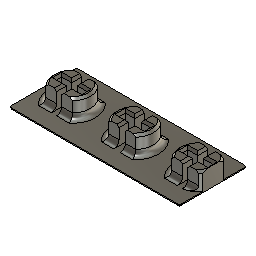
iNTEX_2u_Rotated (Autodesk Fusion 360 design; units mm, degrees)
Autodesk Fusion 360 part; units mm, degrees
sketch "Sketch1" plane through (0, 0, 0) normal (0, 0, 1) x (1, 0, 0)
  line L0 (18.5, 9) -> (-18.5, 9) construction
  line L1 (-18.5, 9) -> (-18.5, -9) construction
  line L2 (-18.5, -9) -> (18.5, -9) construction
  line L3 (18.5, -9) -> (18.5, 9) construction
  line L4 (18.5, 9) -> (-18.5, -9) construction
  line L5 (-18.5, 9) -> (18.5, -9) construction
  line L6 (-17.5, 6.4) -> (14.9, 6.4)
  line L7 (14.9, 6.4) -> (14.9, -6.4)
  line L8 (14.9, -6.4) -> (-17.5, -6.4)
  line L9 (-17.5, -6.4) -> (-17.5, 6.4)
  circle A0 centre (0, 0) radius 3.5
  line L10 (2.4, -0.6) -> (-2.4, -0.6)
  line L11 (-2.4, -0.6) -> (-2.4, 0.6)
  line L12 (-2.4, 0.6) -> (2.4, 0.6)
  line L13 (2.4, 0.6) -> (2.4, -0.6)
  line L14 (2.4, -0.6) -> (-2.4, 0.6) construction
  line L15 (-2.4, -0.6) -> (2.4, 0.6) construction
  line L16 (0.6, -2.4) -> (-0.6, -2.4)
  line L17 (-0.6, -2.4) -> (-0.6, 2.4)
  line L18 (-0.6, 2.4) -> (0.6, 2.4)
  line L19 (0.6, 2.4) -> (0.6, -2.4)
  line L20 (0.6, -2.4) -> (-0.6, 2.4) construction
  line L21 (-0.6, -2.4) -> (0.6, 2.4) construction
  line L22 (-0.6, 2.4) -> (-2.5475, 2.4)
  line L23 (0.6, 2.4) -> (2.5475, 2.4)
  line L24 (-0.6, -2.4) -> (-2.5475, -2.4)
  line L25 (0.6, -2.4) -> (2.5475, -2.4)
  line L26 (0, 0) -> (0, 6.2895) construction
  line L27 (0, 0) -> (12, 0) construction
  circle A1 centre (12, 0) radius 3.5
  line L28 (14.4, -0.5) -> (9.6, -0.5)
  line L29 (9.6, -0.5) -> (9.6, 0.5)
  line L30 (9.6, 0.5) -> (14.4, 0.5)
  line L31 (14.4, 0.5) -> (14.4, -0.5)
  line L32 (14.4, -0.5) -> (9.6, 0.5) construction
  line L33 (9.6, -0.5) -> (14.4, 0.5) construction
  line L34 (12.5, -2.4) -> (11.5, -2.4)
  line L35 (11.5, -2.4) -> (11.5, 2.4)
  line L36 (11.5, 2.4) -> (12.5, 2.4)
  line L37 (12.5, 2.4) -> (12.5, -2.4)
  line L38 (12.5, -2.4) -> (11.5, 2.4) construction
  line L39 (11.5, -2.4) -> (12.5, 2.4) construction
  line L40 (11.5, 2.4) -> (9.4525, 2.4)
  line L41 (12.5, 2.4) -> (14.5475, 2.4)
  line L42 (11.5, -2.4) -> (9.4525, -2.4)
  line L43 (12.5, -2.4) -> (14.5475, -2.4)
  circle A2 centre (-12, 0) radius 3.5
  line L44 (-11.5, 2.4) -> (-9.4525, 2.4)
  line L45 (-11.5, 2.4) -> (-12.5, 2.4)
  line L46 (-12.5, 2.4) -> (-14.5475, 2.4)
  line L47 (-11.5, -2.4) -> (-9.4525, -2.4)
  line L48 (-12.5, -2.4) -> (-11.5, -2.4)
  line L49 (-12.5, -2.4) -> (-14.5475, -2.4)
  line L50 (-11.5, -2.4) -> (-11.5, 2.4)
  line L51 (-12.5, 2.4) -> (-12.5, -2.4)
  line L52 (-14.4, -0.5) -> (-9.6, -0.5)
  line L53 (-9.6, 0.5) -> (-14.4, 0.5)
  line L54 (-14.4, 0.5) -> (-14.4, -0.5)
  line L55 (-9.6, -0.5) -> (-9.6, 0.5)
  point P0 (12, 0)
  point P1 (12, 0)
  dimension "d1" = 37
  dimension "d2" = 18
  dimension "d3" = 2.6
  dimension "d4" = 2.6
  dimension "d5" = 3.6
  dimension "d6" = 1
  dimension "d7" = 7
  dimension "d8" = 4.8
  dimension "d9" = 1.2
  dimension "d10" = 1.2
  dimension "d11" = 4.8
  dimension "d19" = 12
  dimension "d20" = 7
  dimension "d21" = 4.8
  dimension "d22" = 1
  dimension "d23" = 4.8
  dimension "d24" = 1
  constraint perpendicular L0 L1
  constraint parallel L0 L2
  constraint parallel L1 L3
  constraint horizontal L0
  constraint coincident L4 A0.centre
  constraint coincident L5 A0.centre
  constraint coincident A0.centre L26.start
  constraint horizontal L6
  constraint vertical L7
  constraint horizontal L8
  constraint vertical L9
  constraint perpendicular L10 L11
  constraint parallel L10 L12
  constraint parallel L11 L13
  constraint horizontal L10
  constraint coincident L14 A0.centre
  constraint coincident L15 A0.centre
  constraint perpendicular L16 L17
  constraint parallel L16 L18
  constraint parallel L17 L19
  constraint horizontal L16
  constraint coincident L20 A0.centre
  constraint coincident L21 A0.centre
  constraint coincident A0 L22.end
  constraint perpendicular L17 L22
  constraint coincident A0 L23.end
  constraint perpendicular L19 L23
  constraint coincident A0 L24.end
  constraint perpendicular L17 L24
  constraint coincident A0 L25.end
  constraint perpendicular L19 L25
  constraint vertical L26
  constraint perpendicular L19 L27
  constraint coincident P1 P0
  constraint perpendicular L28 L29
  constraint parallel L28 L30
  constraint parallel L29 L31
  constraint horizontal L28
  constraint coincident L32 P1
  constraint coincident L33 P1
  constraint perpendicular L34 L35
  constraint parallel L34 L36
  constraint parallel L35 L37
  constraint horizontal L34
  constraint coincident L38 P1
  constraint coincident L39 P1
  constraint coincident A1 L40.end
  constraint perpendicular L35 L40
  constraint coincident A1 L41.end
  constraint perpendicular L37 L41
  constraint coincident A1 L42.end
  constraint perpendicular L35 L42
  constraint coincident A1 L43.end
  constraint perpendicular L37 L43
  constraint symmetric L26 A1 A2
  constraint symmetric L26 L28.start L52.start
  constraint symmetric L26 L28.end L52.end
  constraint symmetric L26 L29.end L53.start
  constraint symmetric L26 L30.end L53.end
  constraint symmetric L26 L34.start L48.start
  constraint symmetric L26 L34.end L47.start
  constraint symmetric L26 L35.end L44.start
  constraint symmetric L26 L36.end L45.end
  constraint symmetric L26 L40.end L44.end
  constraint symmetric L26 L41.end L46.end
  constraint symmetric L26 L42.end L47.end
  constraint symmetric L26 L43.end L49.end
  measures "d1" distance of L1.end L2.end
  measures "d2" distance of L0.end L1.end
  measures "d3" distance of L2 L8
  measures "d4" distance of L0 L6
  measures "d5" distance of L3 L7
  measures "d6" distance of L1 L9
  measures "d7" diameter of A0
  measures "d8" distance of L11.end L12.end
  measures "d9" distance of L10.end L11.end
  measures "d10" distance of L17.end L18.end
  measures "d11" distance of L16.end L17.end
  measures "d19" distance of A0.centre P1
  measures "d20" diameter of A1
  measures "d21" distance of L29.end L30.end
  measures "d22" distance of L28.end L29.end
  measures "d23" distance of L34.end L35.end
  measures "d24" distance of L35.end L36.end
extrude "Extrude1" add sketch "Sketch1" along normal blind 0.6 contours L6 L7 L8 L9 A1 | L7 A1 L28 L30 L31 L37 L41 L43 | A1 L36 L40 L41 | A1 L34 L42 L43 | A1 L28 L29 L30 L35 L40 L42 | L30 L35 L36 L37 | L28 L34 L35 L37 | L28 L30 L35 L37 | L28 L30 L31 L37 | L28 L29 L30 L35 | A0 L10 L12 L13 L19 L23 L25 | A0 L18 L22 L23 | A0 L16 L24 L25 | A0 L10 L11 L12 L17 L22 L24 | L12 L17 L18 L19 | L10 L16 L17 L19 | L10 L12 L17 L19 | L10 L12 L13 L19 | L10 L11 L12 L17 | A2 L44 L47 L50 L52 L53 L55 | A2 L44 L45 L46 | A2 L47 L48 L49 | A2 L46 L49 L51 L52 L53 L54 | L45 L50 L51 L53 | L48 L50 L51 L52 | L50 L52 L53 L55 | L50 L51 L52 L53 | L51 L52 L53 L54
extrude "Extrude2" add sketch "Sketch1" along normal blind 4 contours L7 A1 L28 L30 L31 L37 L41 L43 | A1 L28 L29 L30 L35 L40 L42 | A0 L10 L12 L13 L19 L23 L25 | A0 L10 L11 L12 L17 L22 L24 | A2 L44 L47 L50 L52 L53 L55 | A2 L46 L49 L51 L52 L53 L54
fillet "Fillet1" radius 1 17 edges at (-1.5738, -2.4, 0.6) (-3.5, 0, 0.6) (1.5738, -2.4, 0.6) (3.5, 0, 0.6) (1.5738, 2.4, 0.6) (-1.5738, 2.4, 0.6) (-10.4762, 2.4, 0.6) (-8.5, 0, 0.6) (-13.5238, 2.4, 0.6) (-15.5, 0, 0.6) (8.5, 0, 0.6) (10.4762, 2.4, 0.6) (13.5238, 2.4, 0.6) (-13.5238, -2.4, 0.6) (-10.4762, -2.4, 0.6) (10.4762, -2.4, 0.6) (13.5238, -2.4, 0.6)
fillet "Fillet1" radius 0.5 4 edges at (14.9, 6.4, 0.3) (-17.5, 6.4, 0.3) (14.9, -6.4, 0.3) (-17.5, -6.4, 0.3)
chamfer "Chamfer1" distance 0.4 angle 45 45 edges at (-1.3, 6.4, 0) (-17.3536, 6.2536, 0) (-17.5, 0, 0) (-17.3536, -6.2536, 0) (-1.3, -6.4, 0) (14.7536, -6.2536, 0) (14.9, 0, 0) (14.7536, 6.2536, 0) (-0.6, 1.5, 4) (-1.5, 0.6, 4) (-2.4, 0, 4) (-1.5, -0.6, 4) (-0.6, -1.5, 4) (0.6, -1.5, 4) (1.5, -0.6, 4) (2.4, 0, 4) (1.5, 0.6, 4) (0.6, 1.5, 4) (3.5, 0, 4) (-3.5, 0, 4) (-12.5, -1.45, 4) (-13.45, -0.5, 4) (-14.4, 0, 4) (-13.45, 0.5, 4) (-12.5, 1.45, 4) (-11.5, 1.45, 4) (-10.55, 0.5, 4) (-9.6, 0, 4) (-10.55, -0.5, 4) (-11.5, -1.45, 4) (-8.5, 0, 4) (-15.5, 0, 4) (8.5, 0, 4) (11.5, 1.45, 4) (10.55, 0.5, 4) (9.6, 0, 4) (10.55, -0.5, 4) (11.5, -1.45, 4) (12.5, -1.45, 4) (13.45, -0.5, 4) (14.4, 0, 4) (13.45, 0.5, 4) (12.5, 1.45, 4) (14.7327, 2.1869, 4) (14.7327, -2.1869, 4)
named bodies: "iNTEX_2u_Rotated"
